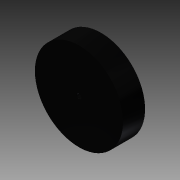
# Autodesk Inventor part: koło
Saved by Autodesk Inventor 2014 (Build 180170000, 170)
## iProperties
Created: 2013-10-14
Part Number: koło
Material: Żywica acetalowa, czarna
Document SubType Name: Modeling
Designer: Wojciech
Density: 1.425 g/cm^3
Appearance: Gładkie - czarne
Author: Wojciech
Autodesk Inventor part; units mm, degrees
ref_plane "YZ Plane" through (0, 0, 0) normal (1, 0, 0) x (0, 1, 0)
ref_plane "XZ Plane" through (0, 0, 0) normal (0, 1, 0) x (-1, 0, 0)
ref_plane "XY Plane" through (0, 0, 0) normal (0, 0, 1) x (1, 0, 0)
sketch "Szkic1" plane through (0, 0, 0) normal (0, 1, 0) x (-1, 0, 0)
  circle A0 centre (0, 0) radius 30
  dimension "d0" = 60
  constraints: 1 centre point, 1 coincident
  measures "d0" diameter of A0
extrude "Wyciągnięcie proste1" add sketch "Szkic1" along normal blind 15
sketch "Szkic2" plane through (0, 15, 0) normal (0, 1, 0) x (1, 0, 0)
  circle A0 centre (0, 0) radius 30 projected
  circle A1 centre (0, 0) radius 1.5
  dimension "d3" = 3
  constraints: 1 centre point, 1 coincident
  measures "d3" diameter of A1
hole "Otwór1" at (0, 15, 0) direction (0, -1, 0) diameter 3 depth 15 tip angle 118
chamfer "Faza1" distance 0.2 angle 45 1 edges at (0, 15, -1.5)
chamfer "Faza2" distance 0.2 angle 45 1 edges at (0, 0, -1.5)
